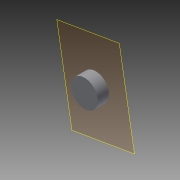
# Autodesk Inventor part: Magnet
Saved by Autodesk Inventor 2014 (Build 180170000, 170)
## iProperties
Created: 2014-01-11
Part Number: Magnet
Material: Generic
Document SubType Name: Modeling
Designer: intern
Density: 1 g/cm^3
Appearance: Default
Author: intern
Autodesk Inventor part; units mm, degrees
ref_plane "YZ Plane" through (0, 0, 0) normal (1, 0, 0) x (0, 1, 0)
ref_plane "XZ Plane" through (0, 0, 0) normal (0, 1, 0) x (-1, 0, 0)
ref_plane "XY Plane" through (0, 0, 0) normal (0, 0, 1) x (1, 0, 0)
ref_plane "Work Plane1" through (26.9875, 590.55, 11.1443) normal (0, 0, 1) x (-0.1684, 0.9857, 0)
sketch "Sketch1" plane through (26.9875, 590.55, 11.1443) normal (0, 0, 1) x (-0.1684, 0.9857, 0)
  circle A0 centre (0, 0) radius 3 projected
  point P0 (-577.5774, 126.0235)
extrude "Extrusion1" add sketch "Sketch1" along normal blind 2.5
body "Solid1"
